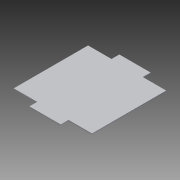
# Autodesk Inventor part: Belly Board
Saved by Autodesk Inventor 2014 SP1 (Build 180222100, 222)
## iProperties
Created: 2014-01-18
Part Number: Belly Board
Material: ABS Plastic
Document SubType Name: Modeling
Designer: Paul
Density: 1.06 g/cm^3
Appearance: Smooth - White
Author: Paul
Autodesk Inventor part; units mm, degrees
ref_plane "YZ Plane" through (0, 0, 0) normal (1, 0, 0) x (0, 1, 0)
ref_plane "XZ Plane" through (0, 0, 0) normal (0, 1, 0) x (-1, 0, 0)
ref_plane "XY Plane" through (0, 0, 0) normal (0, 0, 1) x (1, 0, 0)
sketch "Sketch1" plane through (0, 0, 0) normal (0, 1, 0) x (-1, 0, 0)
  line L0 (0, 0) -> (508, 0)
  line L1 (508, 0) -> (508, 584.2)
  line L2 (508, 584.2) -> (0, 584.2)
  line L3 (0, 584.2) -> (0, 0)
  dimension "d0" = 508
  dimension "d1" = 584.2
  constraints: 8 end point, 2 parallel, 1 horizontal, 1 perpendicular
  measures "d0" distance between parallel lines of L1 L3
  measures "d1" distance of L2.end L0.start
extrude "Extrusion1" add sketch "Sketch1" along normal blind 6.35
sketch "Sketch2" plane through (0, 0, 0) normal (0, -1, 0) x (1, 0, 0)
  line L0 (-508, 584.2) -> (-355.6, 584.2)
  line L1 (-355.6, 584.2) -> (-355.6, 520.7)
  line L2 (-355.6, 520.7) -> (-508, 520.7)
  line L3 (-508, 520.7) -> (-508, 584.2)
  line L4 (0, 584.2) -> (-152.4, 584.2)
  line L5 (-152.4, 584.2) -> (-152.4, 520.7)
  line L6 (-152.4, 520.7) -> (0, 520.7)
  line L7 (0, 520.7) -> (0, 584.2)
  line L8 (-508, 0) -> (-355.6, 0)
  line L9 (-355.6, 0) -> (-355.6, 63.5)
  line L10 (-355.6, 63.5) -> (-508, 63.5)
  line L11 (-508, 63.5) -> (-508, 0)
  line L12 (0, 0) -> (-152.4, 0)
  line L13 (-152.4, 0) -> (-152.4, 63.5)
  line L14 (-152.4, 63.5) -> (0, 63.5)
  line L15 (0, 63.5) -> (0, 0)
  dimension "d4" = 152.4
  dimension "d5" = 63.5
  dimension "d6" = 152.4
  dimension "d7" = 63.5
  dimension "d8" = 152.4
  dimension "d9" = 63.5
  dimension "d10" = 152.4
  dimension "d11" = 63.5
  constraints: 32 end point, 8 parallel, 4 horizontal, 4 perpendicular
  measures "d4" distance of L1.end L2.end
  measures "d5" distance of L0.end L1.end
  measures "d6" distance of L5.end L6.end
  measures "d7" distance of L4.end L5.end
  measures "d8" distance of L9.end L10.end
  measures "d9" distance of L8.end L9.end
  measures "d10" distance of L13.end L14.end
  measures "d11" distance of L12.end L13.end
extrude "Extrusion2" cut sketch "Sketch2" against normal through all
body "Solid1"
